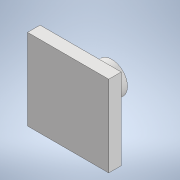
# Autodesk Inventor part: corredor
Saved by Autodesk Inventor 2022 (Build 260153000, 153)
## iProperties
Created: 2022-08-29
Part Number: corredor
Material: Generic
Document SubType Name: Modeling
Designer: cvss2
Density: 1 g/cm^3
Appearance: Default
Author: cvss2
Autodesk Inventor part; units mm, degrees
ref_plane "YZ Plane" through (0, 0, 0) normal (1, 0, 0) x (0, 1, 0)
ref_plane "XZ Plane" through (0, 0, 0) normal (0, 1, 0) x (-1, 0, 0)
ref_plane "XY Plane" through (0, 0, 0) normal (0, 0, 1) x (1, 0, 0)
sketch "Sketch1" plane through (0, 0, 0) normal (0, 0, 1) x (1, 0, 0)
  circle A0 centre (0, 0) radius 2.5
  line L0 (-13, 13) -> (13, 13)
  line L1 (13, 13) -> (13, -13)
  line L2 (13, -13) -> (-13, -13)
  line L3 (-13, -13) -> (-13, 13)
  line L4 (-13, 13) -> (13, -13) construction
  line L5 (13, 13) -> (-13, -13) construction
  dimension "d0" = 5
  dimension "d1" = 26
  dimension "d2" = 26
  constraints: 12 end point, 2 midpoint, 2 parallel, 1 centre point, 1 coincident, 1 horizontal, 1 perpendicular
  measures "d0" diameter of A0
  measures "d1" distance of L1.end L2.end
  measures "d2" distance of L0.end L1.end
extrude "Extrusion1" add sketch "Sketch1" against normal blind 10 contours A0
extrude "Extrusion2" add sketch "Sketch1" along normal blind 4 contours A0 | L0 L1 L2 L3
body "Solid1"
